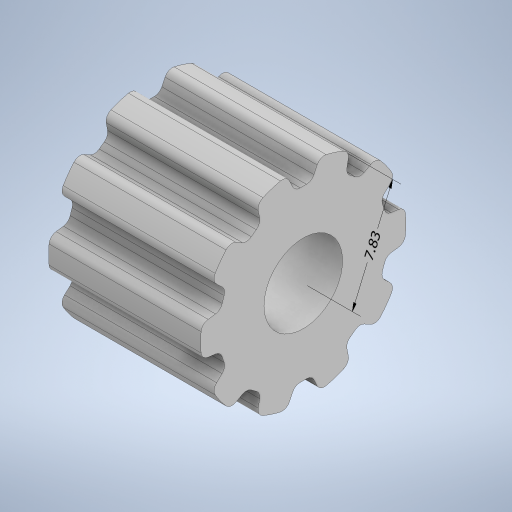
# Autodesk Inventor part: belt_geared_roller_fixed
Saved by Autodesk Inventor 2024.1 (Build 281209000, 209)
## iProperties
Category: PARTsolutions
Company: MISUMI
Created: 2025-03-14
Part Number: belt_geared_roller_fixed
Material: Generic
Catalog Web Link: www.cadenas.de
Description: ATP__XL025, ATP__XL031, ATP__ XL037, ATP__XL050, BTP__XL025, BTP__XL031, BTP__XL037, BTP__XL050, KTP__XL025, KTP__XL031, KTP__ XL037, KTP__XL050, NTP__XL025, NTP__XL031, NTP__ XL037, NTP__XL050, MTP__XL025, MTP__ XL037, MTP__XL050, MTPB__XL025, MTPB__ XL037, MTPB__XL050, MTPP__XL025, MTPP__ XL037, MTPP__XL050, STP__XL025, STP__XL031, STP__ XL037, STP__XL050, KATP__XL025, KATP__XL031, KATP__ XL037, KATP__XL050, KKTP__XL025, KKTP__XL031, KKTP__ XL037, KKTP__XL050_body-Timing Pulleys XL Type
Vendor: MISUMI
Document SubType Name: Modeling
Designer: psAdmin
Manufacturer: MISUMI
Mass: 2.47719 g
Surface Area: 24.0125 cm^2
Volume: 2.47719 cm^3
Density: 1 g/cm^3
Appearance: PSOLRGB-175-175-175
PSOL_IDENT_0: {$CADENAS_DATA/23d-libs/misumi/metric/51_timing_pulleys/mtp_xl/mtp_xl.prj},892 {VTYP=3D},{NB=STP10XL
PSOL_IDENT_1: 025-A-H6.35_b},{LINA=STP10XL025-A-H6.35},{NN=ATP__XL025, ATP__XL031, ATP__ XL037, ATP__XL050, BTP__X
PSOL_IDENT_2: L025, BTP__XL031, BTP__XL037, BTP__XL050, KTP__XL025, KTP__XL031, KTP__ XL037, KTP__XL050, NTP__XL02
PSOL_IDENT_3: 5, NTP__XL031, NTP__ XL037, NTP__XL050, MTP__XL025, MTP__ XL037, MTP__XL050, MTPB__XL025, MTPB__ XL0
PSOL_IDENT_4: 37, MTPB__XL050, MTPP__XL025, MTPP__ XL037, MTPP__XL050, STP__XL025, STP__XL031, STP__ XL037, STP__X
PSOL_IDENT_5: L050, KATP__XL025, KATP__XL031, KATP__ XL037, KATP__XL050, KKTP__XL025, KKTP__XL031, KKTP__ XL037, K
PSOL_IDENT_6: KTP__XL050_body},{DATE=06.01.2023 09:07:12},{GEOMDATE=06.01.2023 09:06:51},{VERSION=},{LINEID=290},{
PSOL_IDENT_7: WBVAR=MATP,ST,TNW,PS,SBS,DD,Z,J,Q,R,S,T,ALT1,ALT2,M,QSC,QFC,QTC,ALT3,K,KSC,KFC,KTC,ALT4,ZM,ZSC,ZFC,Z
PSOL_IDENT_8: TC,ALT5,ALT6,ALT7,FC,ALT8,SRG,ALT9,BTC,TL,ALT10,TPC,ALT11,BC,ALT12,SLH,ALT13,BN},{WBNUMERIC=DD,Z,J,Q
PSOL_IDENT_9: ,R,S,T,QSC,QFC,QTC,K,KSC,KFC,KTC,ZSC,ZFC,ZTC,FC,SRG,BTC,TL,BC,SLH,BN}  {NB=STP10XL025-A-H6.35_b},{LI
PSOL_IDENT_10: NA=STP10XL025-A-H6.35},{KT=DUMMY},{PN=STP10XL025-A-H6.35},{TYPE=STP},{MATP=SUS304},{MATPALG= 'A2017'
PSOL_IDENT_11: ,'Aluminum Alloy 2000 series','S45C','1045 Carbon Steel Equivalent','SUS304','SUS304', 'A6000', '600
PSOL_IDENT_12: 0 Series Aluminum Alloy' },{ST=-},{STALG= '-','-' },{NT=10},{TNW=XL025},{TNWALG= 'XL025','XL031','XL
PSOL_IDENT_13: 037','XL050' },{BW=6.4mm (1/4inch)},{PS=A},{PSALG= 'A','B' },{SBS=H},{SBSALG= 'H','Round Hole','V','
PSOL_IDENT_14: Stepped Hole','Y','Both Ends Stepped Hole','WB','Double Stepped Hole' },{DD=6.35},{DDALG=[4:4/1],4.5
PSOL_IDENT_15: ,[5:6/1],6.35,[7:8/1]},{DDHA=[4:4/1],4.5,[5:6/1],6.35,[7:8/1]},{DDPA=},{DDNA=},{DDNK=[10:10/1]},{DDC
PSOL_IDENT_16: A=},{DDVA=[4:4/1],4.5,[5:6/1]},{DDY=[4:6/1]},{DDWB=[4:4/1]},{DDHB=},{DDPB=},{DDNB=},{DDCB=},{DDVFB=}
PSOL_IDENT_17: ,{Z=0},{ZALG=[0]},{ZMIN=9.000},{ZAMAX=8.000},{ZBMAX=0.000},{DDZ=6.350},{J=0.0},{JALG=[0]},{JMIN=2.00
PSOL_IDENT_18: 0},{JMAX=10.5},{JPN=},{Q=0},{QALG=[0]},{QRMIN=8.350},{QRMAX=8},{WBQMIN=10.350},{R=0},{RALG=[0]},{WBR
PSOL_IDENT_19: MAX=-2.000},{S=0.0},{SALG=[0]},{SMAX=6.5},{T=0.0},{TALG=[0]},{TMAX=8},{SBSPN=-H6.35},{A=7.5},{W=12.5
PSOL_IDENT_20: },{L=0},{PD=16.17},{OD=15.66},{D=0},{DALG=10.000},{DE=12},{F=24},{E=12},{TT=1.6},{BBK=0.000},{TTK=0.
PSOL_IDENT_21: 0},{ALT1=},{ANG=108.000},{ALT1ALG= '','Not applicable' },{ALT1PN=},{ALT2=},{ALT2ALG= '','Not applica
PSOL_IDENT_22: ble' },{M=N/A},{MALG= 'N/A' },{MFTALG= 'N/A' },{MSALG= 'N/A' },{M3D=0.000},{KDML=0.000},{ML=0.000},{
PSOL_IDENT_23: MUL=0.000},{PITCH=0.000},{QSC=0.0},{QSCALG=0},{QFC=0.0},{QFCALG=0},{QTC=0.0},{QTCALG=0},{QPCDMIN=0.0
PSOL_IDENT_24: 00},{QPCDMINALG=0.000},{QPCDMAX=8.000},{ALT2PN=},{TAP=0.000},{ALT3=},{ALT3ALG= '','Not applicable' }
PSOL_IDENT_25: ,{K=0.0},{KALG=0},{KMIN=4.000},{KFTMAX=0.000},{KSMAX=0.000},{KSC=0.0},{KSCALG=0},{KFC=0.0},{KFCALG=0
PSOL_IDENT_26: },{KTC=0.0},{KTCALG=0},{KSCMIN=10.500},{KPCDMIN=10.500},{KPCDMAX=8.000},{ALT3PN=},{ALT4=},{ALT4ALG= ''
PSOL_IDENT_27: ,'Not applicable' },{ALT4MIN=16.850},{ALT4MAX=1.500},{ZM=N/A},{ZMALG= 'N/A' },{ZMFTALG= 'N/A' },{ZMS
PSOL_IDENT_28: ALG= 'N/A' },{ZMDD1=0.0},{ZMDD2=0.0},{ZMHH=0.0},{ZSC=0.0},{ZSCALG=[0]},{ZFC=0.0},{ZFCALG=[0]},{ZTC=0
PSOL_IDENT_29: .0},{ZTCALG=[0]},{ZPCDMIN=0.000},{ZPCDMINALG=0.000},{ZPCDMAX=8.000},{ALT4PN=},{ALT5=},{ALT5ALG= '','
PSOL_IDENT_30: w/o Flange not Attached','NFC','with NFC (Flange not Attached)' },{ALT5PN=},{ALT6=},{ALT6ALG= '','w/
PSOL_IDENT_31: o Flange Attached on One Side Only','RFC','with RFC (Flange Attached on The Boss Side Only)','LFC','
PSOL_IDENT_32: with LFC (Flange Attached on The Opposite Side Only)' },{ALT6PN=},{ALT7=},{ALT7ALG= '','w/o FC (Flan
PSOL_IDENT_33: ge Cut)','FC','with FC (Flange Cut)' },{FC=0.0},{FCALG=0},{FCMIN=17.0},{FCMAX=22.0},{ALT7PN=},{ALT8=
PSOL_IDENT_34: },{ALT8ALG= '','Not applicable' },{ALT8ALGALG=8.000},{ALT8DD2=0.000},{ALT8MM=0.000},{ALT8NN=0.000},{
PSOL_IDENT_35: QC=0.000},{KC=0.000},{ZC=0.000},{SRG=0.0},{SRGALG=[0]},{SRGMAX=0.000},{DD2=0.0},{MM=0.00},{NN=0.00},
PSOL_IDENT_36: {ALT8PN=},{ALT9=},{ALT9ALG= '','Not applicable' },{BTC9=0.000},{TL9=0.000},{BTC=0},{BTCALG=[0]},{TL=
PSOL_IDENT_37: 0.0},{TLALG=0},{TLMIN=0.000},{TLMAX=0.000},{BTCL=0},{BTCD=0},{ALT9PN=},{WLBCTL=12.500},{ALT10=},{ALT
PSOL_IDENT_38: 10ALG= '','Not applicable' },{TPC=N/A},{TPCALG= 'N/A' },{TPCM=4.000},{ALT10PN=},{ALT11=},{ALT11ALG= ''
PSOL_IDENT_39: ,'Not applicable' },{BC=0.0},{BCALG=0},{BCMIN=3},{BCMAX=-13},{M1WBC=6.25},{ALT11PN=},{KTT=4.655},{AL
PSOL_IDENT_40: T12=},{ALT12ALG= '','Not applicable' },{SLHALG=[0]},{SLH=0},{ALT12PN=},{ALT13=},{ALT13ALG= '', 'Not
PSOL_IDENT_41: applicable' },{BN=0.0},{BNALG=0},{BNMIN=-12},{BNMAX=-2.5},{ALT13PN=},{AC=-},{M1=4.000},{M1L=3.000},{
PSOL_IDENT_42: KEYA=0.000},{KEYB=0.000},{KEYM=0.000}
NB: STP10XL025-A-H6.35_b
NN: 0
NT: 10
NBSYN: $PN._b
LINA: STP10XL025-A-H6.35
CATALOG: Misumi
PN: STP10XL025-A-H6.35
MATP: SUS304
ST: -
TNW: XL025
BW: 6.4mm (1/4inch)
PS: A
SBS: Round Hole
DD: 6.35
Z: 0
J: 0
Q: 0
R: 0
S: 0
T: 0
A: 7.5
W: 12.5
L: 0
PD: 16.17
OD: 15.66
D: 0
F: 24
E: 12
TT: 1.6
ALT1: Not applicable
ALT2: Not applicable
M: N/A
QSC: 0
QFC: 0
QTC: 0
ALT3: Not applicable
K: 0
KSC: 0
KFC: 0
KTC: 0
ALT4: Not applicable
ZM: N/A
ZMDD1: 0
ZMDD2: 0
ZMHH: 0
ZSC: 0
ZFC: 0
ZTC: 0
ALT5: w/o Flange not Attached
ALT6: w/o Flange Attached on One Side Only
ALT7: w/o FC (Flange Cut)
FC: 0
ALT8: Not applicable
SRG: 0
DD2: 0
MM: 0
ALT9: Not applicable
BTC: 0
TL: 0
BTCL: 0
BTCD: 0
ALT10: Not applicable
TPC: N/A
ALT11: Not applicable
BC: 0
ALT12: Not applicable
SLH: 0
ALT13: Not applicable
BN: 0
AC: -
SUPPLIER: MISUMI
ARTICLENO: STP10XL025-A-H6.35_b
BOMINFO: STP10XL025-A-H6.35
CREATOR: CADENAS GmbH
Title: STP10XL025-A-H6.35
Author: Cadenas PARTsolutions
Comments: Timing Pulleys XL Type
Autodesk Inventor part; units mm, degrees
ref_plane "YZ Plane" through (0, 0, 0) normal (1, 0, 0) x (0, 1, 0)
ref_plane "XZ Plane" through (0, 0, 0) normal (0, 1, 0) x (-1, 0, 0)
ref_plane "XY Plane" through (0, 0, 0) normal (0, 0, 1) x (1, 0, 0)
sketch "_____2" plane through (0, 0, 0) normal (0, 0, 1) x (1, 0, 0)
  line L0 (12.5, 0) -> (0, 0)
  line L1 (0, 0) -> (0, 6)
  line L2 (0, 6) -> (0.9, 6)
  line L3 (0.9, 6) -> (0.9, 7.619356)
  line L4 (0.9, 7.619356) -> (-0.162829, 11.58589)
  line L5 (-0.162829, 11.58589) -> (1.382652, 12)
  line L6 (1.382652, 12) -> (2.5, 7.83)
  line L7 (2.5, 7.83) -> (10, 7.83)
  line L8 (10, 7.83) -> (11.117348, 12)
  line L9 (11.117348, 12) -> (12.662829, 11.58589)
  line L10 (12.662829, 11.58589) -> (11.6, 7.619356)
  line L11 (11.6, 7.619356) -> (11.6, 6)
  line L12 (11.6, 6) -> (12.5, 6)
  line L13 (12.5, 6) -> (12.5, 0)
  line L14 (12.5, 0) -> (0, 0)
  constraints: 30 end point
revolve "Revolution1" add sketch "_____2" angle 360 about axis through (12.5, 0, 0) along (1, 0, 0)
sketch "Sketch2" plane through (12.5, 0, 0) normal (1, 0, 0) x (0, 0, -1)
  point P0 (0, 0)
hole "Hole1" at (12.5, 0, 0) direction (-1, 0, 0) diameter 6.35 depth 12.5
sketch "_____6" plane through (2.5, 0, 0) normal (1, 0, 0) x (0, 0, -1)
  arc A0 (-8.085, 0) -> (-6.540902, -4.752244) centre (0, 0) ccw
  arc A1 (-6.540902, -4.752244) -> (-2.498402, -7.689292) centre (0, 0) ccw
  arc A2 (-2.498402, -7.689292) -> (2.498402, -7.689292) centre (0, 0) ccw
  arc A3 (2.498402, -7.689292) -> (6.540902, -4.752244) centre (0, 0) ccw
  arc A4 (6.540902, -4.752244) -> (8.085, 0) centre (0, 0) ccw
  arc A5 (8.085, 0) -> (6.540902, 4.752244) centre (0, 0) ccw
  arc A6 (6.540902, 4.752244) -> (2.498402, 7.689292) centre (0, 0) ccw
  arc A7 (2.498402, 7.689292) -> (-2.498402, 7.689292) centre (0, 0) ccw
  arc A8 (-2.498402, 7.689292) -> (-6.540902, 4.752244) centre (0, 0) ccw
  arc A9 (-6.540902, 4.752244) -> (-8.085, 0) centre (0, 0) ccw
  arc A10 (-7.83, 0) -> (-7.798487, -0.701787) centre (0, 0) ccw
  arc A11 (-7.798487, -0.701787) -> (-7.265282, -1.252568) centre (-7.190942, -0.647114) ccw
  line L0 (-7.265282, -1.252568) -> (-6.696552, -1.322399)
  arc A12 (-6.18421, -1.760808) -> (-6.696552, -1.322399) centre (-6.770893, -1.927852) ccw
  arc A13 (-6.18421, -1.760808) -> (-6.038108, -2.210464) centre (0, 0) ccw
  arc A14 (-6.194911, -2.866292) -> (-6.038108, -2.210464) centre (-6.61093, -2.420166) ccw
  line L1 (-6.194911, -2.866292) -> (-6.613977, -3.257077)
  arc A15 (-6.613977, -3.257077) -> (-6.721609, -4.016077) centre (-6.197958, -3.703203) ccw
  arc A16 (-6.721609, -4.016077) -> (-6.334603, -4.602359) centre (0, 0) ccw
  arc A17 (-6.334603, -4.602359) -> (-5.896608, -5.151593) centre (0, 0) ccw
  arc A18 (-5.896608, -5.151593) -> (-5.141496, -5.283774) centre (-5.43723, -4.750256) ccw
  line L2 (-5.141496, -5.283774) -> (-4.640338, -5.005978)
  arc A19 (-3.968154, -5.059511) -> (-4.640338, -5.005978) centre (-4.344604, -5.539496) ccw
  arc A20 (-3.968154, -5.059511) -> (-3.585654, -5.337414) centre (0, 0) ccw
  arc A21 (-3.327025, -5.960156) -> (-3.585654, -5.337414) centre (-3.925817, -5.843762) ccw
  line L3 (-3.327025, -5.960156) -> (-3.436358, -6.522629)
  arc A22 (-3.436358, -6.522629) -> (-3.077305, -7.199937) centre (-2.837566, -6.639023) ccw
  arc A23 (-3.077305, -7.199937) -> (-2.419603, -7.446773) centre (0, 0) ccw
  arc A24 (-2.419603, -7.446773) -> (-1.742425, -7.633666) centre (0, 0) ccw
  arc A25 (-1.742425, -7.633666) -> (-1.053833, -7.296758) centre (-1.606681, -7.038961) ccw
  line L4 (-1.053833, -7.296758) -> (-0.811672, -6.777443)
  arc A26 (-0.236398, -6.425653) -> (-0.811672, -6.777443) centre (-0.258825, -7.035241) ccw
  arc A27 (-0.236398, -6.425653) -> (0.236398, -6.425653) centre (0, 0) ccw
  arc A28 (0.811672, -6.777443) -> (0.236398, -6.425653) centre (0.258825, -7.035241) ccw
  line L5 (0.811672, -6.777443) -> (1.053833, -7.296758)
  arc A29 (1.053833, -7.296758) -> (1.742425, -7.633666) centre (1.606681, -7.038961) ccw
  arc A30 (1.742425, -7.633666) -> (2.419603, -7.446773) centre (0, 0) ccw
  arc A31 (2.419603, -7.446773) -> (3.077304, -7.199937) centre (0, 0) ccw
  arc A32 (3.077304, -7.199937) -> (3.436358, -6.522629) centre (2.837566, -6.639023) ccw
  line L6 (3.436358, -6.522629) -> (3.327025, -5.960156)
  arc A33 (3.585654, -5.337414) -> (3.327025, -5.960156) centre (3.925817, -5.843762) ccw
  arc A34 (3.585654, -5.337414) -> (3.968154, -5.059511) centre (0, 0) ccw
  arc A35 (4.640338, -5.005978) -> (3.968154, -5.059511) centre (4.344604, -5.539496) ccw
  line L7 (4.640338, -5.005978) -> (5.141496, -5.283774)
  arc A36 (5.141496, -5.283774) -> (5.896608, -5.151594) centre (5.43723, -4.750256) ccw
  arc A37 (5.896608, -5.151594) -> (6.334603, -4.602359) centre (0, 0) ccw
  arc A38 (6.334603, -4.602359) -> (6.721609, -4.016077) centre (0, 0) ccw
  arc A39 (6.721609, -4.016077) -> (6.613977, -3.257077) centre (6.197958, -3.703203) ccw
  line L8 (6.613977, -3.257077) -> (6.194911, -2.866292)
  arc A40 (6.038108, -2.210464) -> (6.194911, -2.866292) centre (6.61093, -2.420166) ccw
  arc A41 (6.038108, -2.210464) -> (6.18421, -1.760808) centre (0, 0) ccw
  arc A42 (6.696552, -1.322399) -> (6.18421, -1.760808) centre (6.770893, -1.927852) ccw
  line L9 (6.696552, -1.322399) -> (7.265282, -1.252568)
  arc A43 (7.265282, -1.252568) -> (7.798487, -0.701788) centre (7.190942, -0.647114) ccw
  arc A44 (7.798487, -0.701788) -> (7.83, 0) centre (0, 0) ccw
  arc A45 (7.83, 0) -> (7.798487, 0.701787) centre (0, 0) ccw
  arc A46 (7.798487, 0.701787) -> (7.265282, 1.252568) centre (7.190942, 0.647114) ccw
  line L10 (7.265282, 1.252568) -> (6.696552, 1.322399)
  arc A47 (6.18421, 1.760808) -> (6.696552, 1.322399) centre (6.770893, 1.927852) ccw
  arc A48 (6.18421, 1.760808) -> (6.038108, 2.210464) centre (0, 0) ccw
  arc A49 (6.194911, 2.866292) -> (6.038108, 2.210464) centre (6.61093, 2.420166) ccw
  line L11 (6.194911, 2.866292) -> (6.613977, 3.257077)
  arc A50 (6.613977, 3.257077) -> (6.721609, 4.016077) centre (6.197958, 3.703203) ccw
  arc A51 (6.721609, 4.016077) -> (6.334603, 4.602359) centre (0, 0) ccw
  arc A52 (6.334603, 4.602359) -> (5.896608, 5.151593) centre (0, 0) ccw
  arc A53 (5.896608, 5.151593) -> (5.141496, 5.283774) centre (5.43723, 4.750256) ccw
  line L12 (5.141496, 5.283774) -> (4.640338, 5.005978)
  arc A54 (3.968154, 5.059511) -> (4.640338, 5.005978) centre (4.344604, 5.539496) ccw
  arc A55 (3.968154, 5.059511) -> (3.585654, 5.337414) centre (0, 0) ccw
  arc A56 (3.327025, 5.960156) -> (3.585654, 5.337414) centre (3.925817, 5.843762) ccw
  line L13 (3.327025, 5.960156) -> (3.436358, 6.522629)
  arc A57 (3.436358, 6.522629) -> (3.077305, 7.199937) centre (2.837566, 6.639023) ccw
  arc A58 (3.077305, 7.199937) -> (2.419603, 7.446773) centre (0, 0) ccw
  arc A59 (2.419603, 7.446773) -> (1.742425, 7.633666) centre (0, 0) ccw
  arc A60 (1.742425, 7.633666) -> (1.053833, 7.296758) centre (1.606681, 7.038961) ccw
  line L14 (1.053833, 7.296758) -> (0.811672, 6.777443)
  arc A61 (0.236398, 6.425653) -> (0.811672, 6.777443) centre (0.258825, 7.035241) ccw
  arc A62 (0.236398, 6.425653) -> (-0.236398, 6.425653) centre (0, 0) ccw
  arc A63 (-0.811672, 6.777443) -> (-0.236398, 6.425653) centre (-0.258825, 7.035241) ccw
  line L15 (-0.811672, 6.777443) -> (-1.053833, 7.296758)
  arc A64 (-1.053833, 7.296758) -> (-1.742425, 7.633666) centre (-1.606681, 7.038961) ccw
  arc A65 (-1.742425, 7.633666) -> (-2.419603, 7.446773) centre (0, 0) ccw
  arc A66 (-2.419603, 7.446773) -> (-3.077304, 7.199937) centre (0, 0) ccw
  arc A67 (-3.077304, 7.199937) -> (-3.436358, 6.522629) centre (-2.837566, 6.639023) ccw
  line L16 (-3.436358, 6.522629) -> (-3.327025, 5.960156)
  arc A68 (-3.585654, 5.337414) -> (-3.327025, 5.960156) centre (-3.925817, 5.843762) ccw
  arc A69 (-3.585654, 5.337414) -> (-3.968154, 5.059511) centre (0, 0) ccw
  arc A70 (-4.640338, 5.005978) -> (-3.968154, 5.059511) centre (-4.344604, 5.539496) ccw
  line L17 (-4.640338, 5.005978) -> (-5.141496, 5.283774)
  arc A71 (-5.141496, 5.283774) -> (-5.896608, 5.151594) centre (-5.43723, 4.750256) ccw
  arc A72 (-5.896608, 5.151594) -> (-6.334603, 4.602359) centre (0, 0) ccw
  arc A73 (-6.334603, 4.602359) -> (-6.721609, 4.016077) centre (0, 0) ccw
  arc A74 (-6.721609, 4.016077) -> (-6.613977, 3.257077) centre (-6.197958, 3.703203) ccw
  line L18 (-6.613977, 3.257077) -> (-6.194911, 2.866292)
  arc A75 (-6.038108, 2.210464) -> (-6.194911, 2.866292) centre (-6.61093, 2.420166) ccw
  arc A76 (-6.038108, 2.210464) -> (-6.18421, 1.760808) centre (0, 0) ccw
  arc A77 (-6.696552, 1.322399) -> (-6.18421, 1.760808) centre (-6.770893, 1.927852) ccw
  line L19 (-6.696552, 1.322399) -> (-7.265282, 1.252568)
  arc A78 (-7.265282, 1.252568) -> (-7.798487, 0.701788) centre (-7.190942, 0.647114) ccw
  arc A79 (-7.798487, 0.701788) -> (-7.83, 0) centre (0, 0) ccw
  constraints: 160 point on circle, 80 centre point, 40 end point
extrude "Extrusion1" cut sketch "_____6" along normal blind 7.5
sketch "スケッチ4" plane through (0.9, 0, 0) normal (-1, 0, 0) x (0, 0, 1)
  circle A0 centre (0, 0) radius 12
  circle A1 centre (0, 0) radius 12 projected
  constraints: 1 centre point, 1 coincident, 1 concentric
extrude "押し出し2" cut sketch "スケッチ4" along normal through all
sketch "スケッチ5" plane through (0.9, 0, 0) normal (-1, 0, 0) x (0, 0, 1)
  circle A0 centre (0, 0) radius 9
  circle A1 centre (0, 0) radius 12 projected
  dimension "d12" = 18
  constraints: 1 centre point, 1 coincident
  measures "d12" diameter of A0
extrude "押し出し3" cut sketch "スケッチ5" against normal through all
sketch "スケッチ6" plane through (11.6, 0, 0) normal (1, 0, 0) x (0, 0, -1)
  circle A0 centre (0, 0) radius 9
  constraints: 1 centre point, 1 coincident
extrude "押し出し4" cut sketch "スケッチ6" along normal blind 1.6 and the other way blind 1.6
sketch "スケッチ11" plane through (0.9, 0, 0) normal (-1, 0, 0) x (0, 0, 1)
  circle A0 centre (0, 0) radius 9 projected
  circle A1 centre (0, 0) radius 3.175 projected
extrude "押し出し9" cut sketch "スケッチ11" against normal up to surface (1.6 mm away)
sketch "スケッチ12" plane through (2.5, 0, 0) normal (-1, 0, 0) x (0, 0, 1)
  arc A0 (6.721609, -4.016077) -> (6.613977, -3.257077) centre (6.197958, -3.703203) ccw
  line L0 (6.194911, -2.866292) -> (6.613977, -3.257077)
  arc A1 (6.038108, -2.210464) -> (6.194911, -2.866292) centre (6.61093, -2.420166) ccw
  arc A2 (6.038108, -2.210464) -> (6.18421, -1.760808) centre (0, 0) ccw
  arc A3 (6.696552, -1.322399) -> (6.18421, -1.760808) centre (6.770893, -1.927852) ccw
  line L1 (7.265282, -1.252568) -> (6.696552, -1.322399)
  arc A4 (7.265282, -1.252568) -> (7.798487, -0.701788) centre (7.190942, -0.647115) ccw
  arc A5 (7.798487, -0.701788) -> (7.798487, 0.701788) centre (0, 0) ccw
  arc A6 (7.798487, 0.701788) -> (7.265282, 1.252568) centre (7.190942, 0.647114) ccw
  line L2 (6.696552, 1.322399) -> (7.265282, 1.252568)
  arc A7 (6.18421, 1.760808) -> (6.696552, 1.322399) centre (6.770893, 1.927852) ccw
  arc A8 (6.18421, 1.760808) -> (6.038108, 2.210464) centre (0, 0) ccw
  arc A9 (6.194911, 2.866292) -> (6.038108, 2.210464) centre (6.61093, 2.420166) ccw
  line L3 (6.613977, 3.257077) -> (6.194911, 2.866292)
  arc A10 (6.613977, 3.257077) -> (6.721609, 4.016077) centre (6.197958, 3.703203) ccw
  arc A11 (6.721609, 4.016077) -> (5.896608, 5.151593) centre (0, 0) ccw
  arc A12 (5.896608, 5.151593) -> (5.141496, 5.283774) centre (5.43723, 4.750256) ccw
  line L4 (4.640338, 5.005978) -> (5.141496, 5.283774)
  arc A13 (3.968154, 5.059511) -> (4.640338, 5.005978) centre (4.344604, 5.539496) ccw
  arc A14 (3.968154, 5.059511) -> (3.585654, 5.337414) centre (0, 0) ccw
  arc A15 (3.327025, 5.960156) -> (3.585654, 5.337414) centre (3.925817, 5.843762) ccw
  line L5 (3.436358, 6.522629) -> (3.327025, 5.960156)
  arc A16 (3.436358, 6.522629) -> (3.077304, 7.199937) centre (2.837566, 6.639023) ccw
  arc A17 (3.077304, 7.199937) -> (1.742425, 7.633666) centre (0, 0) ccw
  arc A18 (1.742425, 7.633666) -> (1.053833, 7.296758) centre (1.606681, 7.038961) ccw
  line L6 (0.811672, 6.777443) -> (1.053833, 7.296758)
  arc A19 (0.236398, 6.425653) -> (0.811672, 6.777443) centre (0.258825, 7.035241) ccw
  arc A20 (0.236398, 6.425653) -> (-0.236398, 6.425653) centre (0, 0) ccw
  arc A21 (-0.811672, 6.777443) -> (-0.236398, 6.425653) centre (-0.258825, 7.035241) ccw
  line L7 (-1.053833, 7.296758) -> (-0.811672, 6.777443)
  arc A22 (-1.053833, 7.296758) -> (-1.742425, 7.633666) centre (-1.606681, 7.038961) ccw
  arc A23 (-1.742425, 7.633666) -> (-3.077304, 7.199937) centre (0, 0) ccw
  arc A24 (-3.077304, 7.199937) -> (-3.436358, 6.522629) centre (-2.837566, 6.639023) ccw
  line L8 (-3.327024, 5.960156) -> (-3.436358, 6.522629)
  arc A25 (-3.585654, 5.337414) -> (-3.327024, 5.960156) centre (-3.925817, 5.843763) ccw
  arc A26 (-3.585654, 5.337414) -> (-3.968154, 5.059511) centre (0, 0) ccw
  arc A27 (-4.640338, 5.005978) -> (-3.968154, 5.059511) centre (-4.344604, 5.539496) ccw
  line L9 (-5.141496, 5.283774) -> (-4.640338, 5.005978)
  arc A28 (-5.141496, 5.283774) -> (-5.896608, 5.151593) centre (-5.43723, 4.750256) ccw
  arc A29 (-5.896608, 5.151593) -> (-6.721609, 4.016077) centre (0, 0) ccw
  arc A30 (-6.721609, 4.016077) -> (-6.613977, 3.257077) centre (-6.197958, 3.703203) ccw
  line L10 (-6.194911, 2.866292) -> (-6.613977, 3.257077)
  arc A31 (-6.038108, 2.210464) -> (-6.194911, 2.866292) centre (-6.61093, 2.420166) ccw
  arc A32 (-6.038108, 2.210464) -> (-6.18421, 1.760808) centre (0, 0) ccw
  arc A33 (-6.696552, 1.322399) -> (-6.18421, 1.760808) centre (-6.770893, 1.927852) ccw
  line L11 (-7.265282, 1.252568) -> (-6.696552, 1.322399)
  arc A34 (-7.265282, 1.252568) -> (-7.798487, 0.701788) centre (-7.190942, 0.647115) ccw
  arc A35 (-7.798487, 0.701788) -> (-7.798487, -0.701787) centre (0, 0) ccw
  arc A36 (-7.798487, -0.701787) -> (-7.265282, -1.252568) centre (-7.190942, -0.647114) ccw
  line L12 (-6.696552, -1.322399) -> (-7.265282, -1.252568)
  arc A37 (-6.18421, -1.760808) -> (-6.696552, -1.322399) centre (-6.770893, -1.927852) ccw
  arc A38 (-6.18421, -1.760808) -> (-6.038108, -2.210464) centre (0, 0) ccw
  arc A39 (-6.194911, -2.866292) -> (-6.038108, -2.210464) centre (-6.61093, -2.420166) ccw
  line L13 (-6.613977, -3.257077) -> (-6.194911, -2.866292)
  arc A40 (-6.613977, -3.257077) -> (-6.721609, -4.016077) centre (-6.197958, -3.703203) ccw
  arc A41 (-6.721609, -4.016077) -> (-5.896608, -5.151593) centre (0, 0) ccw
  arc A42 (-5.896608, -5.151593) -> (-5.141496, -5.283774) centre (-5.43723, -4.750256) ccw
  line L14 (-4.640338, -5.005978) -> (-5.141496, -5.283774)
  arc A43 (-3.968154, -5.059511) -> (-4.640338, -5.005978) centre (-4.344604, -5.539496) ccw
  arc A44 (-3.968154, -5.059511) -> (-3.585654, -5.337414) centre (0, 0) ccw
  arc A45 (-3.327025, -5.960156) -> (-3.585654, -5.337414) centre (-3.925817, -5.843762) ccw
  line L15 (-3.436358, -6.522629) -> (-3.327025, -5.960156)
  arc A46 (-3.436358, -6.522629) -> (-3.077304, -7.199937) centre (-2.837566, -6.639023) ccw
  arc A47 (-3.077304, -7.199937) -> (-1.742425, -7.633666) centre (0, 0) ccw
  arc A48 (-1.742425, -7.633666) -> (-1.053833, -7.296758) centre (-1.606681, -7.038961) ccw
  line L16 (-0.811672, -6.777443) -> (-1.053833, -7.296758)
  arc A49 (-0.236398, -6.425653) -> (-0.811672, -6.777443) centre (-0.258825, -7.035241) ccw
  arc A50 (-0.236398, -6.425653) -> (0.236398, -6.425653) centre (0, 0) ccw
  arc A51 (0.811672, -6.777443) -> (0.236398, -6.425653) centre (0.258825, -7.035241) ccw
  line L17 (1.053833, -7.296758) -> (0.811672, -6.777443)
  arc A52 (1.053833, -7.296758) -> (1.742425, -7.633666) centre (1.606681, -7.038961) ccw
  arc A53 (1.742425, -7.633666) -> (3.077304, -7.199937) centre (0, 0) ccw
  arc A54 (3.077304, -7.199937) -> (3.436358, -6.522629) centre (2.837566, -6.639023) ccw
  line L18 (3.327024, -5.960156) -> (3.436358, -6.522629)
  arc A55 (3.585654, -5.337414) -> (3.327024, -5.960156) centre (3.925817, -5.843763) ccw
  arc A56 (3.585654, -5.337414) -> (3.968154, -5.059511) centre (0, 0) ccw
  arc A57 (4.640338, -5.005978) -> (3.968154, -5.059511) centre (4.344604, -5.539496) ccw
  line L19 (5.141496, -5.283774) -> (4.640338, -5.005978)
  arc A58 (5.141496, -5.283774) -> (5.896608, -5.151593) centre (5.43723, -4.750256) ccw
  arc A59 (5.896608, -5.151593) -> (6.721609, -4.016077) centre (0, 0) ccw
  circle A60 centre (0, 0) radius 3.175
extrude "押し出し10" add sketch "スケッチ12" against normal blind 11.6
sketch "スケッチ13" plane through (2.5, 0, 0) normal (-1, 0, 0) x (0, 0, 1)
  circle A0 centre (0, 0) radius 3
  circle A1 centre (0, 0) radius 3.175 projected
  dimension "d37" = 6
  constraints: 1 centre point, 1 coincident
  measures "d37" diameter of A0
extrude "押し出し11" add sketch "スケッチ13" against normal up to surface (11.6 mm away)
sketch "スケッチ14" plane through (2.5, 0, 0) normal (-1, 0, 0) x (0, 0, 1)
  circle A0 centre (0, 0) radius 1.6
  circle A1 centre (0, 0) radius 3 projected
  dimension "d40" = 3.2
  constraints: 1 centre point, 1 coincident
  measures "d40" diameter of A0
extrude "押し出し12" add sketch "スケッチ14" against normal blind 4.45
body "Solid1"
